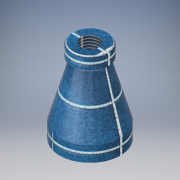
# Autodesk Inventor part: C
Saved by Autodesk Inventor 2017 (Build 210142000, 142)
## iProperties
Part Number: C
Material: 一般
Document SubType Name: Modeling
Designer: user
Density: 1 g/cm^3
Appearance: 1.5 英吋正方形 - 中藍色
Author: user
Autodesk Inventor part; units mm, degrees
ref_plane "YZ Plane" through (0, 0, 0) normal (1, 0, 0) x (0, 1, 0)
ref_plane "XZ Plane" through (0, 0, 0) normal (0, 1, 0) x (-1, 0, 0)
ref_plane "XY Plane" through (0, 0, 0) normal (0, 0, 1) x (1, 0, 0)
sketch "草圖1" plane through (0, 0, 0) normal (0, 0, 1) x (1, 0, 0)
  line L0 (0, 0) -> (20, 0)
  line L1 (20, 0) -> (20, 10)
  line L2 (20, 10) -> (10, 45)
  line L3 (12, 47) -> (10, 45)
  line L4 (12, 47) -> (12, 54)
  line L5 (11, 55) -> (0, 55)
  line L6 (12, 54) -> (11, 55)
  line L7 (0, 0) -> (0, 55)
  point P0 (12, 55)
  dimension "d0" = 20
  dimension "d1" = 10
  dimension "d4" = 8
  dimension "d5" = 1
  dimension "d6" = 45
  dimension "d7" = 2
  dimension "d8" = 2
  dimension "d9" = 55
  dimension "d10" = 10
  constraints: 16 end point, 2 perpendicular, 2 point on line, 2 vertical, 1 horizontal
  measures "d0" distance of L0.start L0.end
  measures "d1" distance of L0.end L1.end
  measures "d4" distance of L3.start point (12, 55)
  measures "d5" distance of L4.end point (12, 55)
  measures "d6" angle of L4 L6
  measures "d7" horizontal distance of L3.start L2.end
  measures "d8" horizontal distance of L3.start L2.end
  measures "d9" distance between parallel lines of L5 L0
  measures "d10" horizontal distance of L2.end L0.start
revolve "迴轉1" add sketch "草圖1" angle 360 about axis through (0, 0, 0) along (0, 1, 0)
sketch "草圖2" plane through (0, 0, 0) normal (0, 0, 1) x (1, 0, 0)
  line L0 (0, 0) -> (15, 0)
  line L1 (-20, 0) -> (20, 0) projected
  line L2 (15, 0) -> (6, 33)
  line L3 (6, 33) -> (0, 33)
  line L4 (0, 33) -> (0, 0)
  dimension "d12" = 15
  dimension "d13" = 6
  dimension "d14" = 33
  constraints: 8 end point, 1 parallel, 1 perpendicular, 1 point on line
  measures "d12" distance of L0.start L0.end
  measures "d13" distance of L2.end L3.end
  measures "d14" distance between parallel lines of L3 L0
revolve "迴轉2" cut sketch "草圖2" angle 360 about axis through (0, 33, 0) along (0, -1, 0)
sketch "草圖3" plane through (0, 33, 0) normal (0, -1, 0) x (1, 0, 0)
  circle A0 centre (0, 0) radius 6
  dimension "d16" = 12
  constraints: 1 centre point, 1 coincident
  measures "d16" diameter of A0
extrude "擠出1" cut sketch "草圖3" against normal through all
thread "螺紋1" size "M12x1.75" class "6H" standard "ANSI Metric M Profile" full length
